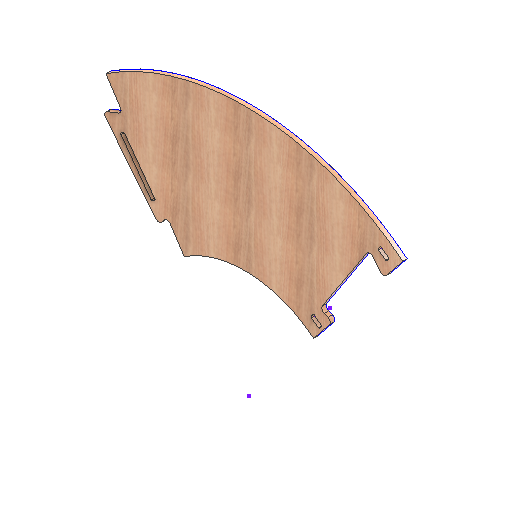
# Autodesk Inventor part: Platform F3
Saved by Autodesk Inventor 2021 (Build 250183000, 183)
## iProperties
Created: 2020-05-09
Part Number: Platform F3
Material: Wood (Birch)
Document SubType Name: Modeling
Designer: Dan Wikman
Density: 0.55 g/cm^3
Appearance: Birch - Natural Polished
Mass: 5289.03 g
Surface Area: 11405 cm^2
Volume: 9616.42 cm^3
Autodesk Inventor part; units mm, degrees
ref_plane "YZ Plane" through (0, 0, 0) normal (1, 0, 0) x (0, 1, 0)
ref_plane "XZ Plane" through (0, 0, 0) normal (0, 1, 0) x (-1, 0, 0)
ref_plane "XY Plane" through (0, 0, 0) normal (0, 0, 1) x (1, 0, 0)
sketch "CONTOURS" plane through (0, 0, 0) normal (0, 0, 1) x (1, 0, 0)
  arc A0 (1467.8843, 188.4261) -> (1444.4964, 189.5904) centre (1455.765, 180.4653) ccw
  line L0 (1444.4964, 189.5904) -> (1433.8001, 176.3815)
  arc A1 (1409.6695, 176.43) -> (1433.8001, 176.3815) centre (1421.7543, 186.136) ccw
  line L1 (1409.6695, 176.43) -> (1205.1516, 431.0714)
  arc A2 (1211.6817, 455.248) -> (1205.1516, 431.0714) centre (1217.2364, 440.7775) ccw
  line L2 (1211.6817, 455.248) -> (1259.5115, 473.6081)
  arc A3 (1259.5115, 473.6081) -> (1266.4344, 495.1059) centre (1254.3152, 487.1451) ccw
  line L3 (1266.4344, 495.1059) -> (1206.4511, 586.4222)
  arc A4 (2416.4096, 529.2878) -> (1206.4511, 586.4222) centre (1772.0714, -275.6668) ccw
  line L4 (2416.4096, 529.2878) -> (2348.9296, 445.0595)
  arc A5 (2326.3448, 445.0004) -> (2348.9296, 445.0595) centre (2337.6134, 454.1255) ccw
  line L5 (2326.3448, 445.0004) -> (2294.0217, 484.916)
  arc A6 (2294.0217, 484.916) -> (2269.0106, 483.6555) centre (2281.976, 475.1615) ccw
  line L6 (2269.0106, 483.6555) -> (2088.6011, 208.2752)
  arc A7 (2088.6011, 208.2752) -> (2096.0118, 185.3107) centre (2101.5665, 199.7812) ccw
  line L7 (2096.0118, 185.3107) -> (2111.7592, 179.2658)
  arc A8 (2117.8791, 156.6628) -> (2111.7592, 179.2658) centre (2106.5629, 165.7289) ccw
  line L8 (2117.8791, 156.6628) -> (2053.1174, 75.8275)
  arc A9 (2053.1174, 75.8275) -> (1525.5022, 100.7107) centre (1772.1395, -275.8029) ccw
  line L9 (1525.5022, 100.7107) -> (1467.8843, 188.4261)
  constraints: 20 end point, 20 point on circle, 10 centre point
sketch "HOLES" plane through (0, 0, 0) normal (0, 0, 1) x (1, 0, 0)
  line L0 (2054.9481, 158.6603) -> (2084.0727, 137.5)
  arc A0 (2084.9576, 131.9128) -> (2084.0727, 137.5) centre (2081.7215, 134.264) ccw
  line L1 (2084.9576, 131.9128) -> (2078.492, 123.0136)
  arc A1 (2072.9048, 122.1287) -> (2078.492, 123.0136) centre (2075.2559, 125.3648) ccw
  line L2 (2072.9048, 122.1287) -> (2043.7801, 143.289)
  arc A2 (2042.8952, 148.8762) -> (2043.7801, 143.289) centre (2046.1313, 146.5251) ccw
  line L3 (2042.8952, 148.8762) -> (2049.3609, 157.7754)
  arc A3 (2054.9481, 158.6603) -> (2049.3609, 157.7754) centre (2052.5969, 155.4242) ccw
  line L4 (1405.0745, 238.9064) -> (1396.1753, 232.4408)
  arc A4 (1390.5881, 233.3257) -> (1396.1753, 232.4408) centre (1393.8242, 235.6768) ccw
  line L5 (1390.5881, 233.3257) -> (1267.741, 402.4102)
  arc A5 (1268.6259, 407.9975) -> (1267.741, 402.4102) centre (1270.9771, 404.7614) ccw
  line L6 (1268.6259, 407.9975) -> (1277.5251, 414.4631)
  arc A6 (1283.1123, 413.5782) -> (1277.5251, 414.4631) centre (1279.8762, 411.227) ccw
  line L7 (1283.1123, 413.5782) -> (1405.9594, 244.4936)
  arc A7 (1405.0745, 238.9064) -> (1405.9594, 244.4936) centre (1402.7234, 242.1425) ccw
  line L8 (2316.1678, 525.0037) -> (2322.6335, 533.9029)
  arc A8 (2328.2207, 534.7878) -> (2322.6335, 533.9029) centre (2325.8696, 531.5518) ccw
  line L9 (2328.2207, 534.7878) -> (2357.3453, 513.6276)
  arc A9 (2358.2302, 508.0403) -> (2357.3453, 513.6276) centre (2354.9942, 510.3915) ccw
  line L10 (2358.2302, 508.0403) -> (2351.7646, 499.1412)
  arc A10 (2346.1774, 498.2562) -> (2351.7646, 499.1412) centre (2348.5285, 501.4923) ccw
  line L11 (2346.1774, 498.2562) -> (2317.0528, 519.4165)
  arc A11 (2316.1678, 525.0037) -> (2317.0528, 519.4165) centre (2319.4039, 522.6526) ccw
  constraints: 24 end point, 24 point on circle, 12 centre point
sketch "LETTERS" plane through (0, 0, 0) normal (0, 0, 1) x (1, 0, 0)
  line L0 (2123.0862, 379.0631) -> (2113.6777, 384.09)
  line L1 (2105.5346, 377.443) -> (2118.4889, 370.5215)
  line L2 (2118.4889, 370.5215) -> (2127.8234, 387.992)
  constraints: 6 end point
extrude "Extrusion3" add sketch "CONTOURS" along normal blind 18
extrude "Extrusion4" cut sketch "HOLES" along normal blind 18
body "Solid1"
